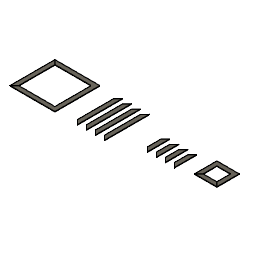
Flanges (Autodesk Fusion 360 design; units mm, degrees)
part number: 2025-11-29-13-37-30-032
Autodesk Fusion 360 part; units mm, degrees
sketch "Sketch1" plane through (0, 0, 0) normal (0, 0, 1) x (1, 0, 0)
  line L0 (-125, 250) -> (-125, -250)
  line L1 (-125, -250) -> (-175, -200)
  line L2 (-175, -200) -> (-175, 200)
  line L3 (-175, 200) -> (-125, 250)
  line L4 (-225, -250) -> (-275, -200)
  line L5 (-275, -200) -> (-275, 200)
  line L6 (-225, 250) -> (-225, -250)
  line L7 (-275, 200) -> (-225, 250)
  line L8 (-325, -250) -> (-375, -200)
  line L9 (-375, -200) -> (-375, 200)
  line L10 (-325, 250) -> (-325, -250)
  line L11 (-375, 200) -> (-325, 250)
  line L12 (-425, -250) -> (-475, -200)
  line L13 (-475, -200) -> (-475, 200)
  line L14 (-425, 250) -> (-425, -250)
  line L15 (-475, 200) -> (-425, 250)
  line L16 (-725, 200) -> (-675, 250)
  line L17 (-675, 250) -> (-675, -250)
  line L18 (-725, -200) -> (-725, 200)
  line L19 (-675, -250) -> (-725, -200)
  line L20 (-725, -200) -> (-675, -250)
  line L21 (-675, -250) -> (-1175, -250)
  line L22 (-1125, -200) -> (-725, -200)
  line L23 (-1175, -250) -> (-1125, -200)
  line L24 (-1174.9614, 249.8579) -> (-1124.9614, 199.8579)
  line L25 (-1124.9614, 199.8579) -> (-1124.9614, -200.1421)
  line L26 (-1174.9614, -250.1421) -> (-1174.9614, 249.8579)
  line L27 (-1124.9614, -200.1421) -> (-1174.9614, -250.1421)
  line L28 (-1125, 200) -> (-1175, 250)
  line L29 (-1175, 250) -> (-675, 250)
  line L30 (-725, 200) -> (-1125, 200)
  line L31 (-675, 250) -> (-725, 200)
  line L32 (225, 125) -> (225, -125)
  line L33 (225, -125) -> (175, -75)
  line L34 (175, -75) -> (175, 75)
  line L35 (175, 75) -> (225, 125)
  line L36 (275, 75) -> (325, 125)
  line L37 (325, 125) -> (325, -125)
  line L38 (275, -75) -> (275, 75)
  line L39 (325, -125) -> (275, -75)
  line L40 (375, -75) -> (375, 75)
  line L41 (425, 125) -> (425, -125)
  line L42 (375, 75) -> (425, 125)
  line L43 (425, -125) -> (375, -75)
  line L44 (475, 75) -> (525, 125)
  line L45 (525, 125) -> (525, -125)
  line L46 (475, -75) -> (475, 75)
  line L47 (525, -125) -> (475, -75)
  line L48 (694.8673, -75.0205) -> (744.8673, -25.0205)
  line L49 (895, -25) -> (895, 125)
  line L50 (745, 125) -> (695, 175)
  line L51 (895, 125) -> (745, 125)
  line L52 (944.8673, -75.0205) -> (694.8673, -75.0205)
  line L53 (945, 175) -> (895, 125)
  line L54 (744.8673, -25.0205) -> (894.8673, -25.0205)
  line L55 (894.8673, -25.0205) -> (944.8673, -75.0205)
  line L56 (895, 125) -> (945, 175)
  line L57 (945, 175) -> (945, -75)
  line L58 (945, -75) -> (895, -25)
  line L59 (695, -75) -> (695, 175)
  line L60 (695, 175) -> (745, 125)
  line L61 (745, 125) -> (745, -25)
  line L62 (695, 175) -> (945, 175)
  line L63 (745, -25) -> (695, -75)
  constraint vertical L0
  constraint parallel L0 L2
  constraint perpendicular L1 L3
  constraint vertical L6
  constraint parallel L5 L6
  constraint perpendicular L4 L7
  constraint vertical L10
  constraint parallel L9 L10
  constraint perpendicular L8 L11
  constraint vertical L14
  constraint parallel L13 L14
  constraint perpendicular L12 L15
  constraint vertical L17
  constraint parallel L17 L18
  constraint perpendicular L16 L19
  constraint parallel L21 L22
  constraint perpendicular L20 L23
  constraint parallel L25 L26
  constraint perpendicular L24 L27
  constraint parallel L29 L30
  constraint perpendicular L28 L31
  constraint vertical L32
  constraint parallel L32 L34
  constraint perpendicular L33 L35
  constraint vertical L37
  constraint parallel L37 L38
  constraint perpendicular L36 L39
  constraint vertical L41
  constraint parallel L40 L41
  constraint perpendicular L42 L43
  constraint vertical L45
  constraint parallel L45 L46
  constraint perpendicular L44 L47
  constraint parallel L52 L54
  constraint perpendicular L48 L55
  constraint parallel L59 L61
  constraint perpendicular L60 L63
  constraint parallel L51 L62
  constraint perpendicular L50 L53
  constraint vertical L57
  constraint parallel L49 L57
  constraint perpendicular L56 L58
extrude "Extrude1" add sketch "Sketch1" along normal blind 4 contours L0 L1 L2 L3 | L4 L5 L6 L7 | L8 L9 L10 L11 | L12 L13 L14 L15 | L16 L28 L29 L30 L31 | L16 L17 L18 L19 L20 L31 | L19 L20 L21 L22 L25 L27 | L22 L23 L24 L25 L26 | L32 L33 L34 L35 | L36 L37 L38 L39 | L40 L41 L42 L43 | L44 L45 L46 L47 | L48 L52 L54 L55 L59 L63 | L48 L50 L54 L59 L60 L61 L63 | L50 L51 L53 L56 L60 L62 | L49 L53 L56 L57 L58 makes body 3 at (-691.6667, -66.6667, 0) makes body 3 at (-1158.3076, -66.7012, 0) makes body 6 at (844.9115, -58.347, 0) makes body 6 at (795, 158.3333, 0) makes body 9 at (-141.6667, -66.6667, 0) makes body 4 at (-241.6667, -66.6667, 0) makes body 2 at (-341.6667, -66.6667, 0) makes body 8 at (-441.6667, -66.6667, 0) makes body 7 at (208.3333, 25, 0) makes body 1 at (308.3333, 25, 0) makes body 5 at (408.3333, 25, 0) makes body 10 at (508.3333, 25, 0)
